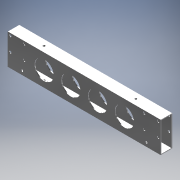
# Autodesk Inventor part: Extrusion Mid
Saved by Autodesk Inventor 2019.4 (Build 234330000, 330)
## iProperties
Created: 2020-01-07
Part Number: Extrusion Mid
Material: Aluminum 6061
Document SubType Name: Modeling
Designer: Mark
Mass: 540.845 g
Surface Area: 1399.55 cm^2
Volume: 200.313 cm^3
Density: 2.7 g/cm^3
Appearance: Aluminum - Flat
Author: Mark
Autodesk Inventor part; units mm, degrees
ref_plane "YZ Plane" through (0, 0, 0) normal (1, 0, 0) x (0, 1, 0)
ref_plane "XZ Plane" through (0, 0, 0) normal (0, 1, 0) x (-1, 0, 0)
ref_plane "XY Plane" through (0, 0, 0) normal (0, 0, 1) x (1, 0, 0)
sketch "Sketch1" plane through (0, 0, 0) normal (1, 0, 0) x (0, 1, 0)
  line L0 (-40, 15) -> (40, 15)
  line L1 (40, 15) -> (40, -15)
  line L2 (40, -15) -> (-40, -15)
  line L3 (-40, -15) -> (-40, 15)
  line L4 (-40, 15) -> (40, -15) construction
  line L5 (40, 15) -> (-40, -15) construction
  line L6 (-38, 13) -> (38, 13)
  line L7 (38, 13) -> (38, -13)
  line L8 (38, -13) -> (-38, -13)
  line L9 (-38, -13) -> (-38, 13)
  line L10 (-38, 13) -> (38, -13) construction
  line L11 (38, 13) -> (-38, -13) construction
  point P0 (0, 0)
  dimension "d0" = 80
  dimension "d1" = 30
  dimension "d2" = 76
  dimension "d3" = 26
  constraints: 24 end point, 4 midpoint, 4 parallel, 2 horizontal, 2 perpendicular
  measures "d0" distance of L1.end L2.end
  measures "d1" distance of L0.end L1.end
  measures "d2" distance of L7.end L8.end
  measures "d3" distance of L6.end L7.end
extrude "Extrusion1" add sketch "Sketch1" along normal blind 400
sketch "Sketch2" plane through (0, -40, -15) normal (0, -1, 0) x (1, 0, 0)
  circle A0 centre (80, 15) radius 2.75
  circle A1 centre (320, 15) radius 2.75
  line L0 (0, 30) -> (400, 30) projected
  line L1 (400, 30) -> (400, 0) projected
  line L2 (0, 0) -> (0, 30) projected
  point P0 (0, 15)
  dimension "d6" = 5.5
  dimension "d7" = 5.5
  dimension "d8" = 15
  dimension "d9" = 80
  dimension "d10" = 15
  dimension "d11" = 80
  constraints: 2 centre point
  measures "d6" diameter of A0
  measures "d7" diameter of A1
  measures "d8" distance from line of L0 A1.centre
  measures "d9" distance from line of L1 A1.centre
  measures "d10" distance from line of L0 A0.centre
  measures "d11" distance from line of L2 A0.centre
extrude "Extrusion2" cut sketch "Sketch2" against normal blind 80
sketch "Sketch3" plane through (0, -40, -15) normal (0, 0, -1) x (-1, 0, 0)
  circle A0 centre (-37.5, 10) radius 2.75
  circle A1 centre (-362.5, 10) radius 2.75
  line L0 (0, 80) -> (-400, 80) projected
  line L1 (-400, 0) -> (-400, 80) projected
  line L2 (0, 80) -> (0, 0) projected
  point P0 (0, 40)
  dimension "d14" = 5.5
  dimension "d15" = 5.5
  dimension "d16" = 70
  dimension "d17" = 37.5
  dimension "d18" = 37.5
  dimension "d19" = 70
  constraints: 2 centre point
  measures "d14" diameter of A0
  measures "d15" diameter of A1
  measures "d16" distance from line of L0 A1.centre
  measures "d17" distance from line of L1 A1.centre
  measures "d18" distance from line of L2 A0.centre
  measures "d19" distance from line of L0 A0.centre
extrude "Extrusion3" cut sketch "Sketch3" against normal blind 30
sketch "Sketch4" plane through (0, -40, -15) normal (0, 0, -1) x (-1, 0, 0)
  line L0 (-43.5, 36.5) -> (-6.5, 36.5) construction
  line L1 (-6.5, 36.5) -> (-6.5, 73.5) construction
  line L2 (-6.5, 73.5) -> (-43.5, 73.5) construction
  line L3 (-43.5, 73.5) -> (-43.5, 36.5) construction
  line L4 (-43.5, 36.5) -> (-6.5, 73.5) construction
  line L5 (-6.5, 36.5) -> (-43.5, 73.5) construction
  circle A0 centre (-6.5, 73.5) radius 3.25
  circle A1 centre (-6.5, 36.5) radius 3.25
  circle A2 centre (-43.5, 73.5) radius 3.25
  circle A3 centre (-43.5, 36.5) radius 3.25
  line L6 (0, 80) -> (0, 0) projected
  line L7 (0, 80) -> (-400, 80) projected
  line L8 (0, 0) -> (-400, 0) projected
  line L9 (-200, 0) -> (-200, 80)
  line L10 (-200, 0) -> (-120, 0) construction
  circle A4 centre (-393.5, 73.5) radius 3.25
  circle A5 centre (-393.5, 36.5) radius 3.25
  circle A6 centre (-356.5, 73.5) radius 3.25
  circle A7 centre (-356.5, 36.5) radius 3.25
  point P0 (0, 40)
  point P1 (-25, 55)
  dimension "d22" = 37
  dimension "d23" = 37
  dimension "d24" = 6.5
  dimension "d25" = 6.5
  dimension "d26" = 6.5
  dimension "d27" = 6.5
  dimension "d28" = 6.5
  dimension "d29" = 6.5
  dimension "d32" = 90
  constraints: 16 end point, 8 centre point, 4 coincident, 4 midpoint, 4 symmetric about line, 2 horizontal, 2 parallel, 2 perpendicular, 4 other
  measures "d22" distance of L2.end L1.end
  measures "d23" distance of L1.end L0.end
  measures "d24" diameter of A0
  measures "d25" diameter of A1
  measures "d26" diameter of A2
  measures "d27" diameter of A3
  measures "d28" distance between parallel lines of L1 L6
  measures "d29" distance between parallel lines of L7 L2
  measures "d32" angle of L10 L9
extrude "Extrusion4" cut sketch "Sketch4" against normal blind 30 contours A0 | A1 | A2 | A3 | A4 | A5 | A6 | A7
sketch "Sketch5" plane through (0, -40, -15) normal (0, 0, -1) x (-1, 0, 0)
  circle A0 centre (-95, 40) radius 25
  line L0 (0, 80) -> (-400, 80) projected
  line L1 (0, 80) -> (0, 0) projected
  circle A1 centre (-165, 40) radius 25
  circle A2 centre (-235, 40) radius 25
  circle A3 centre (-305, 40) radius 25
  point P0 (0, 40)
  dimension "d33" = 50
  dimension "d34" = 40
  dimension "d35" = 95
  dimension "d38" = 70
  constraints: 4 centre point, 1 horizontal, 6 other
  measures "d33" diameter of A0
  measures "d34" distance from line of L0 A0.centre
  measures "d35" distance from line of L1 A0.centre
  measures "d38" distance of A0.centre A1.centre
extrude "Extrusion5" cut sketch "Sketch5" against normal blind 30
body "Solid1"
